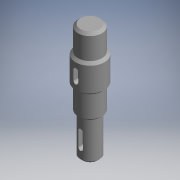
# Autodesk Inventor part: Вал 1,3 (окончание тип 2)
Saved by Autodesk Inventor 2018.1 (Build 221171000, 171)
## iProperties
Part Number: Вал 1,3 (окончание тип 2)
Material: Generic
Document SubType Name: Modeling
Designer: Dmitry
Appearance: Generic
Author: Dmitry
Autodesk Inventor part; units mm, degrees
ref_plane "YZ Plane" through (0, 0, 0) normal (1, 0, 0) x (0, 1, 0)
ref_plane "XZ Plane" through (0, 0, 0) normal (0, 1, 0) x (-1, 0, 0)
ref_plane "XY Plane" through (0, 0, 0) normal (0, 0, 1) x (1, 0, 0)
sketch "Sketch1" plane through (0, 0, 0) normal (0, 0, 1) x (1, 0, 0)
  line L0 (0, 0) -> (20, 0)
  line L1 (20, 0) -> (20, 80)
  line L2 (20, 80) -> (25, 80)
  line L3 (25, 80) -> (25, 130)
  line L4 (25, 130) -> (30, 130)
  line L5 (30, 130) -> (30, 190)
  line L6 (30, 190) -> (25, 190)
  line L7 (25, 190) -> (25, 240)
  line L8 (25, 240) -> (0, 240)
  line L9 (0, 240) -> (0, 0)
  line L10 (0, -48) -> (0, 288) projected
  constraints: 20 end point
revolve "Revolution1" add sketch "Sketch1" angle 360 about axis through (0, -10, 0) along (0, 1, 0)
sketch "Sketch2" plane through (0, 0, 20) normal (0, 0, 1) x (1, 0, 0)
  line L0 (-5, 55) -> (-5, 25)
  line L1 (5, 25) -> (5, 55)
  arc A0 (5, 55) -> (-5, 55) centre (0, 55) ccw
  arc A1 (-5, 25) -> (5, 25) centre (0, 25) ccw
  constraints: 4 end point, 4 point on circle, 2 centre point
extrude "Extrusion1" cut sketch "Sketch2" against normal blind 10
sketch "Sketch3" plane through (0, 0, -25) normal (0, 0, 1) x (1, 0, 0)
  line L0 (5, 112.5) -> (5, 97.5)
  line L1 (-5, 97.5) -> (-5, 112.5)
  arc A0 (5, 112.5) -> (-5, 112.5) centre (0, 112.5) ccw
  arc A1 (-5, 97.5) -> (5, 97.5) centre (0, 97.5) ccw
  line L2 (5, 222.5) -> (5, 207.5)
  line L3 (-5, 207.5) -> (-5, 222.5)
  arc A2 (5, 222.5) -> (-5, 222.5) centre (0, 222.5) ccw
  arc A3 (-5, 207.5) -> (5, 207.5) centre (0, 207.5) ccw
  constraints: 8 end point, 8 point on circle, 4 centre point
extrude "Extrusion2" cut sketch "Sketch3" along normal blind 10
sketch "Sketch4" plane through (0, 0, 30) normal (0, 0, 1) x (1, 0, 0)
  line L0 (-5, 170) -> (-5, 150)
  line L1 (5, 150) -> (5, 170)
  arc A0 (5, 170) -> (-5, 170) centre (0, 170) ccw
  arc A1 (-5, 150) -> (5, 150) centre (0, 150) ccw
  constraints: 4 end point, 4 point on circle, 2 centre point
extrude "Extrusion3" cut sketch "Sketch4" against normal blind 10
chamfer "Chamfer1" distance 5 angle 45 5 edges at (-20, 0, 0) (-25, 80, 0) (-30, 130, 0) (-30, 190, 0) (-25, 240, 0)
body "Solid1"
